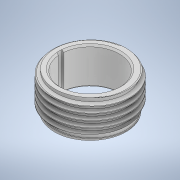
# Autodesk Inventor part: 76. Шестерня спидометра ведущая
Saved by Autodesk Inventor 2021 (Build 250183000, 183)
## iProperties
Created: 2021-03-19
Part Number: 76. Шестерня спидометра ведущая
Material: Типовые
Document SubType Name: Modeling
Designer: Данил
Density: 1 g/cm^3
Appearance: По умолчанию
Author: Данил
Autodesk Inventor part; units mm, degrees
ref_plane "YZ Plane" through (0, 0, 0) normal (1, 0, 0) x (0, 1, 0)
ref_plane "XZ Plane" through (0, 0, 0) normal (0, 1, 0) x (-1, 0, 0)
ref_plane "XY Plane" through (0, 0, 0) normal (0, 0, 1) x (1, 0, 0)
sketch "Эскиз1" plane through (0, 0, 0) normal (0, 0, 1) x (1, 0, 0)
  line L0 (0, 11) -> (0, -11)
  line L1 (18.5, 11) -> (21.5, 11)
  line L2 (21.5, 11) -> (21.5, -11)
  line L3 (21.5, -11) -> (18.5, -11)
  line L4 (17.5, -10) -> (17.5, 10)
  line L5 (17.5, -10) -> (18.5, -11)
  line L6 (17.5, 10) -> (18.5, 11)
  point P0 (0, 0)
  point P1 (0, 0)
  point P2 (17.5, 11)
  point P3 (17.5, -11)
  dimension "d0" = 22
  dimension "d1" = 43
  dimension "d2" = 35
  dimension "d3" = 1
  dimension "d4" = 45
  dimension "d5" = 1
  dimension "d6" = 45
  constraints: 14 end point, 4 point on line, 2 horizontal alignment, 2 parallel, 1 coincident, 1 horizontal, 1 midpoint, 1 perpendicular, 1 vertical
  measures "d0" distance of L0.start L0.end
  measures "d1" diameter of L2 L0
  measures "d2" diameter of L4 L0
  measures "d3" distance of L4.start point (17.5, -11)
  measures "d4" angle of L4 L5
  measures "d5" distance of L4.end point (17.5, 11)
  measures "d6" angle of L4 L6
revolve "Вращение1" add sketch "Эскиз1" angle 360 about axis through (0, 11, 0) along (0, -1, 0)
sketch "Эскиз2" plane through (0, 11, 0) normal (0, 1, 0) x (1, 0, 0)
  circle A0 centre (-0.4984, -0.0405) radius 18
  circle A1 centre (0, 0) radius 17.5 projected
  line L0 (-17.4356, 1.5) -> (-18.4323, 1.5)
  line L1 (-17.4356, -1.5) -> (-18.4391, -1.5)
  circle A2 centre (0, 0) radius 18.5 construction
  point P0 (0, 0)
  dimension "d8" = 36
  dimension "d9" = 3
  dimension "d10" = 1.5
  constraints: 4 end point, 4 point on circle, 2 horizontal, 1 centre point, 1 tangent, 2 other
  measures "d8" diameter of A0
  measures "d9" distance between parallel lines of L1 L0
  measures "d10" distance from line of point (0, 0) L0
extrude "Выдавливание1" cut sketch "Эскиз2" against normal through all both and the other way through all contours A0 L0 A1 L1
sketch "Эскиз3" plane through (0, 0, 0) normal (1, 0, 0) x (0, 1, 0)
  line L0 (11, -21.5) -> (-11, -21.5) projected
  line L1 (11, 21.5) -> (11, -21.5) projected
  line L2 (11, -21.5) -> (8.5, -23.44)
  line L3 (8.5, -23.44) -> (-6.5, -23.44)
  line L4 (-6.5, -23.44) -> (-7.6201, -21.5)
  line L5 (0, 0) -> (11, 0)
  dimension "d22" = 15
  dimension "d23" = 46.88
  dimension "d24" = 30
  dimension "d25" = 2.5
  constraints: 8 end point, 1 horizontal, 1 midpoint, 1 point on line
  measures "d22" distance of L2.end L3.end
  measures "d23" diameter of L3 L5
  measures "d24" angle of L1 L4
  measures "d25" horizontal distance of L0.start L2.end
revolve "Вращение2" add sketch "Эскиз3" angle 360 about axis through (0, 0, 0) along (0, 1, 0)
ref_plane "РабПлоскость1" through (0, -6.5, -23.44) normal (-0.999676, -0.0254538, 0) x (0.0254538, -0.999676, 0)
sketch "Эскиз5" plane through (0, -6.5, -23.44) normal (-0.999676, -0.0254538, 0) x (0.0254538, -0.999676, 0)
  arc A0 (-1.65, 0) -> (-1.15, 2.44) centre (-7.3536, 2.44) ccw
  arc A1 (1.15, 2.44) -> (1.65, 0) centre (7.3536, 2.44) ccw
  line L0 (1.65, 0) -> (-1.65, 0)
  line L1 (-1.15, 2.44) -> (1.15, 2.44)
  point P0 (-6.4979, 23.44)
  point P1 (0, 0)
  point P2 (0, 1.94)
  point P3 (0, 0)
  point P4 (4.4985, 1.94)
  dimension "d48" = 3.3
  dimension "d50" = 2.3
  dimension "d59" = 0.5
  constraints: 4 end point, 4 point on circle, 2 centre point, 2 coincident, 2 horizontal, 2 line through centre, 1 equal radius, 1 horizontal alignment, 1 midpoint, 1 vertical alignment
  measures "d48" distance of L0.start L0.end
  measures "d50" distance of L1.end L1.start
  measures "d59" distance from line of point (0, 1.94) L1
sketch3d "3D эскиз4"
  helix H0 starts at (0, 8.5, -23.44) axis through (0, 8.5, 0) along (0, -1, 0) pitch 3.75 turns 4 hand left
sweep "Сдвиг2" cut profiles "Эскиз5" path "3D эскиз4"
pattern_linear "Прямоуг.массив5" count 2 spacing 15 along (0, -1, 0) of "Сдвиг2"
pattern_linear "Прямоуг.массив6" count 2 spacing 15 along (0, 1, 0) of "Сдвиг2"
equation "\"d5\" = d3"
equation "\"d6\" = d4"
